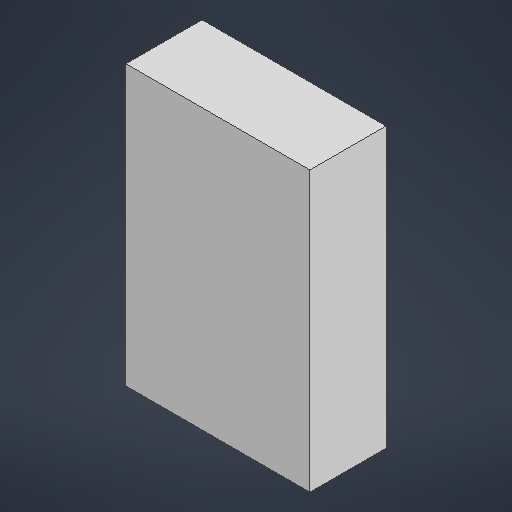
# Autodesk Inventor part: paletas
Saved by Autodesk Inventor 2025.3 (Build 293356000, 356)
## iProperties
Created: 2025-10-20
Part Number: paletas
Material: Generic
Document SubType Name: Modeling
Designer: sophi
Density: 1 g/cm^3
Appearance: Default
Author: sophi
Autodesk Inventor part; units mm, degrees
ref_plane "YZ Plane" through (0, 0, 0) normal (1, 0, 0) x (0, 1, 0)
ref_plane "XZ Plane" through (0, 0, 0) normal (0, 1, 0) x (-1, 0, 0)
ref_plane "XY Plane" through (0, 0, 0) normal (0, 0, 1) x (1, 0, 0)
sketch "Sketch1" plane through (0, 0, 0) normal (0, 1, 0) x (-1, 0, 0)
  line L0 (14.5, 7.0797) -> (0, 7.0797)
  line L1 (0, 7.0797) -> (0, 1.0797)
  line L2 (0, 1.0797) -> (14.5, 1.0797)
  line L3 (14.5, 1.0797) -> (14.5, 7.0797)
  point P0 (0, 0)
  dimension "d0" = 14.5
  dimension "d1" = 6
  constraints: 8 end point, 2 parallel, 1 horizontal, 1 perpendicular, 1 point on line
  measures "d0" distance of L1.end L2.end
  measures "d1" distance of L2.end L0.start
extrude "Extrusion1" add sketch "Sketch1" along normal blind 22
body "Solid1"
